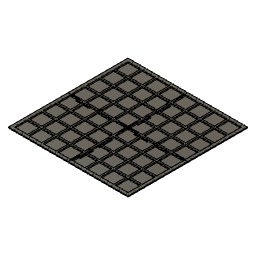
šachovnice v5 v1 (Autodesk Fusion 360 design; units mm, degrees)
Autodesk Fusion 360 part; units mm, degrees
sketch "Sketch1" plane through (0, 0, 0) normal (0, 0, 1) x (1, 0, 0)
  line L0 (-146.9, 146.9) -> (146.9, 146.9)
  line L1 (146.9, 146.9) -> (146.9, -146.9)
  line L2 (146.9, -146.9) -> (-146.9, -146.9)
  line L3 (-146.9, -146.9) -> (-146.9, 146.9)
  line L4 (-111.9, 146.9) -> (-111.9, -146.9) construction
  line L5 (-146.9, 111.9) -> (146.9, 111.9) construction
  line L6 (-74.6, 146.9) -> (-74.6, -146.9) construction
  line L7 (-37.3, 146.9) -> (-37.3, -146.9) construction
  line L8 (0, 146.9) -> (0, -146.9) construction
  line L9 (37.3, 146.9) -> (37.3, -146.9) construction
  line L10 (74.6, 146.9) -> (74.6, -146.9) construction
  line L11 (111.9, 146.9) -> (111.9, -146.9) construction
  line L12 (-146.9, 74.6) -> (146.9, 74.6) construction
  line L13 (-146.9, 37.3) -> (146.9, 37.3) construction
  line L14 (-146.9, 0) -> (146.9, 0) construction
  line L15 (-146.9, -37.3) -> (146.9, -37.3) construction
  line L16 (-146.9, -74.6) -> (146.9, -74.6) construction
  line L17 (-146.9, -111.9) -> (146.9, -111.9) construction
  line L18 (-113.9, 146.9) -> (-113.9, -146.9)
  line L19 (-76.6, 146.9) -> (-76.6, -146.9)
  line L20 (-39.3, 146.9) -> (-39.3, -146.9)
  line L21 (-2, 146.9) -> (-2, -146.9)
  line L22 (35.3, 146.9) -> (35.3, -146.9)
  line L23 (72.6, 146.9) -> (72.6, -146.9)
  line L24 (109.9, 146.9) -> (109.9, -146.9)
  line L25 (-146.9, 109.9) -> (146.9, 109.9)
  line L26 (-146.9, 113.9) -> (146.9, 113.9)
  line L27 (-109.9, 146.9) -> (-109.9, -146.9)
  line L28 (-72.6, 146.9) -> (-72.6, -146.9)
  line L29 (-35.3, 146.9) -> (-35.3, -146.9)
  line L30 (2, 146.9) -> (2, -146.9)
  line L31 (39.3, 146.9) -> (39.3, -146.9)
  line L32 (76.6, 146.9) -> (76.6, -146.9)
  line L33 (113.9, 146.9) -> (113.9, -146.9)
  line L34 (-146.9, 76.6) -> (146.9, 76.6)
  line L35 (-146.9, 72.6) -> (146.9, 72.6)
  line L36 (-146.9, 39.3) -> (146.9, 39.3)
  line L37 (-146.9, 35.3) -> (146.9, 35.3)
  line L38 (-146.9, 2) -> (146.9, 2)
  line L39 (-146.9, -2) -> (146.9, -2)
  line L40 (-146.9, -35.3) -> (146.9, -35.3)
  line L41 (-146.9, -39.3) -> (146.9, -39.3)
  line L42 (-146.9, -72.6) -> (146.9, -72.6)
  line L43 (-146.9, -76.6) -> (146.9, -76.6)
  line L44 (-146.9, -109.9) -> (146.9, -109.9)
  line L45 (-146.9, -113.9) -> (146.9, -113.9)
  line L46 (150.9, -150.9) -> (-150.9, -150.9)
  line L47 (-150.9, -150.9) -> (-150.9, 150.9)
  line L48 (-150.9, 150.9) -> (150.9, 150.9)
  line L49 (150.9, 150.9) -> (150.9, -150.9)
  line L50 (-154.9, -154.9) -> (-154.9, 154.9)
  line L51 (-154.9, 154.9) -> (154.9, 154.9)
  line L52 (154.9, 154.9) -> (154.9, -154.9)
  line L53 (154.9, -154.9) -> (-154.9, -154.9)
  dimension "d8" = 37.3
  dimension "d9" = 0
  dimension "d14" = 0
  dimension "d15" = -37.3
  dimension "d21" = -8
  dimension "d30" = 2
  dimension "d31" = -2
  dimension "d32" = 2
  dimension "d33" = -2
  dimension "d35" = 35
  dimension "d36" = 35
  constraint horizontal L0
  constraint vertical L1
  constraint horizontal L2
  constraint vertical L3
  constraint equal L0 L3
  constraint coincident L0 L4.start
  constraint coincident L2 L4.end
  constraint perpendicular L2 L4
  constraint coincident L3 L5.start
  constraint coincident L1 L5.end
  constraint perpendicular L1 L5
  constraint midpoint L8 origin
  constraint coincident L1 L26.end
  constraint coincident L1 L25.end
  constraint coincident L3 L26.start
  constraint coincident L3 L25.start
  constraint coincident L0 L18.start
  constraint coincident L0 L27.start
  constraint coincident L14 origin
  constraint coincident L8 origin
  measures "d35" distance of L3 L4
  measures "d36" distance of L0 L5
extrude "Extrude1" add sketch "Sketch1" along normal blind 4 contours L0 L18 L26 L27 | L3 L18 L25 L26 | L18 L25 L26 L27 | L0 L19 L26 L28 | L19 L25 L26 L27 | L18 L25 L27 L34 | L3 L18 L34 L35 | L19 L25 L26 L28 | L18 L27 L34 L35 | L0 L20 L26 L29 | L20 L25 L26 L28 | L19 L25 L28 L34 | L19 L27 L34 L35 | L18 L27 L35 L36 | L3 L18 L36 L37 | L20 L25 L26 L29 | L19 L28 L34 L35 | L18 L27 L36 L37 | L0 L21 L26 L30 | L21 L25 L26 L29 | L20 L25 L29 L34 | L20 L28 L34 L35 | L19 L28 L35 L36 | L19 L27 L36 L37 | L18 L27 L37 L38 | L3 L18 L38 L39 | L21 L25 L26 L30 | L20 L29 L34 L35 | L19 L28 L36 L37 | L18 L27 L38 L39 | L0 L22 L26 L31 | L22 L25 L26 L30 | L21 L25 L30 L34 | L21 L29 L34 L35 | L20 L29 L35 L36 | L20 L28 L36 L37 | L19 L28 L37 L38 | L19 L27 L38 L39 | L18 L27 L39 L40 | L3 L18 L40 L41 | L22 L25 L26 L31 | L21 L30 L34 L35 | L20 L29 L36 L37 | L19 L28 L38 L39 | L18 L27 L40 L41 | L0 L23 L26 L32 | L23 L25 L26 L31 | L22 L25 L31 L34 | L22 L30 L34 L35 | L21 L30 L35 L36 | L21 L29 L36 L37 | L20 L29 L37 L38 | L20 L28 L38 L39 | L19 L28 L39 L40 | L19 L27 L40 L41 | L18 L27 L41 L42 | L3 L18 L42 L43 | L23 L25 L26 L32 | L22 L31 L34 L35 | L21 L30 L36 L37 | L20 L29 L38 L39 | L19 L28 L40 L41 | L18 L27 L42 L43 | L0 L24 L26 L33 | L24 L25 L26 L32 | L23 L25 L32 L34 | L23 L31 L34 L35 | L22 L31 L35 L36 | L22 L30 L36 L37 | L21 L30 L37 L38 | L21 L29 L38 L39 | L20 L29 L39 L40 | L20 L28 L40 L41 | L19 L28 L41 L42 | L19 L27 L42 L43 | L18 L27 L43 L44 | L3 L18 L44 L45 | L24 L25 L26 L33 | L23 L32 L34 L35 | L22 L31 L36 L37 | L21 L30 L38 L39 | L20 L29 L40 L41 | L19 L28 L42 L43 | L18 L27 L44 L45 | L1 L25 L26 L33 | L24 L25 L33 L34 | L24 L32 L34 L35 | L23 L32 L35 L36 | L23 L31 L36 L37 | L22 L31 L37 L38 | L22 L30 L38 L39 | L21 L30 L39 L40 | L21 L29 L40 L41 | L20 L29 L41 L42 | L20 L28 L42 L43 | L19 L28 L43 L44 | L19 L27 L44 L45 | L2 L18 L27 L45 | L24 L33 L34 L35 | L23 L32 L36 L37 | L22 L31 L38 L39 | L21 L30 L40 L41 | L20 L29 L42 L43 | L19 L28 L44 L45 | L1 L33 L34 L35 | L24 L33 L35 L36 | L24 L32 L36 L37 | L23 L32 L37 L38 | L23 L31 L38 L39 | L22 L31 L39 L40 | L22 L30 L40 L41 | L21 L30 L41 L42 | L21 L29 L42 L43 | L20 L29 L43 L44 | L20 L28 L44 L45 | L2 L19 L28 L45 | L24 L33 L36 L37 | L23 L32 L38 L39 | L22 L31 L40 L41 | L21 L30 L42 L43 | L20 L29 L44 L45 | L1 L33 L36 L37 | L24 L33 L37 L38 | L24 L32 L38 L39 | L23 L32 L39 L40 | L23 L31 L40 L41 | L22 L31 L41 L42 | L22 L30 L42 L43 | L21 L30 L43 L44 | L21 L29 L44 L45 | L2 L20 L29 L45 | L24 L33 L38 L39 | L23 L32 L40 L41 | L22 L31 L42 L43 | L21 L30 L44 L45 | L1 L33 L38 L39 | L24 L33 L39 L40 | L24 L32 L40 L41 | L23 L32 L41 L42 | L23 L31 L42 L43 | L22 L31 L43 L44 | L22 L30 L44 L45 | L2 L21 L30 L45 | L24 L33 L40 L41 | L23 L32 L42 L43 | L22 L31 L44 L45 | L1 L33 L40 L41 | L24 L33 L41 L42 | L24 L32 L42 L43 | L23 L32 L43 L44 | L23 L31 L44 L45 | L2 L22 L31 L45 | L24 L33 L42 L43 | L23 L32 L44 L45 | L1 L33 L42 L43 | L24 L33 L43 L44 | L24 L32 L44 L45 | L2 L23 L32 L45 | L24 L33 L44 L45 | L1 L33 L44 L45 | L2 L24 L33 L45 | L46 L47 L48 L49 | L50 L51 L52 L53 makes body 1
extrude "Extrude2" add sketch "Sketch1" along normal blind 1 contours L0 L3 L18 L26 | L0 L19 L26 L27 | L3 L18 L25 L34 | L0 L20 L26 L28 | L19 L25 L27 L34 | L3 L18 L35 L36 | L0 L21 L26 L29 | L20 L25 L28 L34 | L19 L27 L35 L36 | L3 L18 L37 L38 | L0 L22 L26 L30 | L21 L25 L29 L34 | L20 L28 L35 L36 | L19 L27 L37 L38 | L3 L18 L39 L40 | L0 L23 L26 L31 | L22 L25 L30 L34 | L21 L29 L35 L36 | L20 L28 L37 L38 | L19 L27 L39 L40 | L3 L18 L41 L42 | L0 L24 L26 L32 | L23 L25 L31 L34 | L22 L30 L35 L36 | L21 L29 L37 L38 | L20 L28 L39 L40 | L19 L27 L41 L42 | L3 L18 L43 L44 | L0 L1 L26 L33 | L24 L25 L32 L34 | L23 L31 L35 L36 | L22 L30 L37 L38 | L21 L29 L39 L40 | L20 L28 L41 L42 | L19 L27 L43 L44 | L2 L3 L18 L45 | L1 L25 L33 L34 | L24 L32 L35 L36 | L23 L31 L37 L38 | L22 L30 L39 L40 | L21 L29 L41 L42 | L20 L28 L43 L44 | L2 L19 L27 L45 | L1 L33 L35 L36 | L24 L32 L37 L38 | L23 L31 L39 L40 | L22 L30 L41 L42 | L21 L29 L43 L44 | L2 L20 L28 L45 | L1 L33 L37 L38 | L24 L32 L39 L40 | L23 L31 L41 L42 | L22 L30 L43 L44 | L2 L21 L29 L45 | L1 L33 L39 L40 | L24 L32 L41 L42 | L23 L31 L43 L44 | L2 L22 L30 L45 | L1 L33 L41 L42 | L24 L32 L43 L44 | L2 L23 L31 L45 | L1 L33 L43 L44 | L2 L24 L32 L45 | L1 L2 L33 L45 bodies 1
extrude "Extrude3" cut sketch "Sketch1" along normal blind 2 contours L50 L51 L52 L53 bodies 1
sketch "Sketch2" plane through (0, 0, 0) normal (0, 0, -1) x (1, 0, 0)
  line L0 (-150.9, 150.9) -> (-150.9, -150.9)
  line L1 (-150.9, -150.9) -> (150.9, -150.9)
  line L2 (150.9, -150.9) -> (150.9, 150.9)
  line L3 (150.9, 150.9) -> (-150.9, 150.9)
sketch "Sketch3" plane through (0, 0, 0) normal (0, 0, 1) x (-1, 0, 0)
  line L0 (154.9, -154.9) -> (154.9, 154.9)
  line L1 (-5, -105.4443) -> (-5, -70) construction
  line L2 (5, -130.4443) -> (5, -95.4443) construction
  line L3 (0, -125.4443) -> (5, -130.4443) construction
  line L4 (-5, -55) -> (-5, -20) construction
  line L5 (5, -80) -> (5, -45) construction
  line L6 (-5, 45) -> (-5, 80) construction
  line L7 (5, 20) -> (5, 55) construction
  line L8 (-5, 130) -> (0, 125) construction
  line L9 (-5, 95) -> (-5, 130) construction
  line L10 (5, 70) -> (5, 105) construction
  line L11 (5.1, -130.6857) -> (5.1, -95.2029)
  line L12 (-4.9, -105.2029) -> (-4.9, -70.2414)
  line L13 (5.1, -80.2414) -> (5.1, -44.7586)
  line L14 (-4.9, -54.7586) -> (-4.9, -20.2414)
  line L15 (5.1, 19.7586) -> (5.1, 55.2414)
  line L16 (-4.9, 45.2414) -> (-4.9, 79.7586)
  line L17 (5.1, 69.7586) -> (5.1, 105.2414)
  line L18 (-4.9, 95.2414) -> (-4.9, 129.7586)
  line L19 (4.9, -130.2029) -> (4.9, -95.6857)
  line L20 (-5.1, -105.6857) -> (-5.1, -69.7586)
  line L21 (4.9, -79.7586) -> (4.9, -45.2414)
  line L22 (-5.1, -55.2414) -> (-5.1, -19.7586)
  line L23 (4.9, 20.2414) -> (4.9, 54.7586)
  line L24 (-5.1, 44.7586) -> (-5.1, 80.2414)
  line L25 (4.9, 70.2414) -> (4.9, 104.7586)
  line L26 (-5.1, 94.7586) -> (-5.1, 130.2414)
  line L27 (55, -5) -> (20, -5) construction
  line L28 (79.7586, 4.9) -> (45.2414, 4.9)
  line L29 (80, 5) -> (45, 5) construction
  line L30 (-44.7586, -5.1) -> (-80.2414, -5.1)
  line L31 (-95.0618, -4.9) -> (-129.5789, -4.9)
  line L32 (-45.2414, -4.9) -> (-79.7586, -4.9)
  line L33 (80.2414, 5.1) -> (44.7586, 5.1)
  line L34 (130.2414, 5.1) -> (94.7586, 5.1)
  line L35 (-19.7586, 5.1) -> (-55.2414, 5.1)
  line L36 (-20, 5) -> (-55, 5) construction
  line L37 (105, -5) -> (70, -5) construction
  line L38 (54.7586, -4.9) -> (20.2414, -4.9)
  line L39 (55.2414, -5.1) -> (19.7586, -5.1)
  line L40 (-20.2414, 4.9) -> (-54.7586, 4.9)
  line L41 (105.2414, -5.1) -> (69.7586, -5.1)
  line L42 (-94.8203, -5) -> (-129.8203, -5) construction
  line L43 (104.7586, -4.9) -> (70.2414, -4.9)
  line L44 (130, 5) -> (95, 5) construction
  line L45 (-45, -5) -> (-80, -5) construction
  line L46 (-69.6687, 5.1898) -> (-105.1516, 5.1898)
  line L47 (-94.5789, -5.1) -> (-130.0618, -5.1)
  line L48 (-70.1516, 4.9898) -> (-104.6687, 4.9898)
  line L49 (-69.9102, 5.0898) -> (-104.9102, 5.0898) construction
  line L50 (129.7586, 4.9) -> (95.2414, 4.9)
  line L51 (-129.8203, -5) -> (-124.8203, 0) construction
  line L52 (20, -5) -> (25, 0) construction
  line L53 (19.7586, -5.1) -> (24.7586, -0.1)
  line L54 (25, 0) -> (0, 0) construction
  line L55 (25.2414, 0.1) -> (0, 0.1)
  line L56 (24.7586, -0.1) -> (0, -0.1)
  line L57 (-20, 5) -> (-25, 0) construction
  line L58 (-19.7586, 5.1) -> (-24.7586, 0.1)
  line L59 (-24.7586, 0.1) -> (0, 0.1)
  line L60 (-25, 0) -> (0, 0) construction
  line L61 (-20.2414, 4.9) -> (-25.2414, -0.1)
  line L62 (0, -0.1) -> (-25.2414, -0.1)
  line L63 (-5, -20) -> (0, -25) construction
  line L64 (0, -25) -> (0, 0) construction
  line L65 (-5.1, -19.7586) -> (-0.1, -24.7586)
  line L66 (-0.1, -24.7586) -> (-0.1, -0.1)
  line L67 (-4.9, -20.2414) -> (0.1, -25.2414)
  line L68 (0.1, -25.2414) -> (0.1, -0.1)
  line L69 (5, 20) -> (0, 25) construction
  line L70 (0, 25) -> (0, 0) construction
  line L71 (5.1, 19.7586) -> (0.1, 24.7586)
  line L72 (0.1, 24.7586) -> (0.1, 0.1)
  line L73 (4.9, 20.2414) -> (-0.1, 25.2414)
  line L74 (-0.1, 25.2414) -> (-0.1, 0.1)
  line L75 (-124.8203, 0) -> (-157, 0) construction
  line L76 (-124.5789, 0.1) -> (-157, 0.1)
  line L77 (-130.0618, -5.1) -> (-125.0618, -0.1)
  line L78 (-125.0618, -0.1) -> (-157, -0.1)
  line L79 (0, 125) -> (0, 163.2119) construction
  line L80 (-5.1, 130.2414) -> (-0.1, 125.2414)
  line L81 (-0.1, 125.2414) -> (-0.1, 156.7338)
  line L82 (0.1, 124.7586) -> (0.1, 159.9994)
  line L83 (130, 5) -> (125, 0) construction
  line L84 (125, 0) -> (175, 0) construction
  line L85 (130.2414, 5.1) -> (125.2414, 0.1)
  line L86 (125.2414, 0.1) -> (175.0792, 0.1)
  line L87 (129.7586, 4.9) -> (124.7586, -0.1)
  line L88 (124.7586, -0.1) -> (175.0791, -0.1)
  line L89 (0, -125.4443) -> (0, -160) construction
  line L90 (-0.1, -125.2029) -> (-0.1, -160)
  line L91 (5.1, -130.6857) -> (0.1, -125.6857)
  line L92 (0.1, -125.6857) -> (0.1, -160)
  line L93 (5.1, 55.2414) -> (-4.9, 45.2414)
  line L94 (4.9, 54.7586) -> (-5.1, 44.7586)
  line L95 (5, 55) -> (-5, 45) construction
  line L96 (5, 70) -> (-5, 80) construction
  line L97 (4.9, 70.2414) -> (-5.1, 80.2414)
  line L98 (5.1, 69.7586) -> (-4.9, 79.7586)
  line L99 (4.9, 104.7586) -> (-5.1, 94.7586)
  line L100 (5, 105) -> (-5, 95) construction
  line L101 (5.1, 105.2414) -> (-4.9, 95.2414)
  line L102 (0.1, 124.7586) -> (-4.9, 129.7586)
  line L103 (-55, 5) -> (-45, -5) construction
  line L104 (-45.2414, -4.9) -> (-55.2414, 5.1)
  line L105 (-54.7586, 4.9) -> (-44.7586, -5.1)
  line L106 (-69.9102, 5.0898) -> (-80, -5) construction
  line L107 (-70.1516, 4.9898) -> (-80.2414, -5.1)
  line L108 (-69.6687, 5.1898) -> (-79.7586, -4.9)
  line L109 (-94.8203, -5) -> (-104.9102, 5.0898) construction
  line L110 (-105.1516, 5.1898) -> (-95.0618, -4.9)
  line L111 (-104.6687, 4.9898) -> (-94.5789, -5.1)
  line L112 (-124.5789, 0.1) -> (-129.5789, -4.9)
  line L113 (5, -45) -> (-5, -55) construction
  line L114 (4.9, -45.2414) -> (-5.1, -55.2414)
  line L115 (5.1, -44.7586) -> (-4.9, -54.7586)
  line L116 (5, -80) -> (-5, -70) construction
  line L117 (4.9, -79.7586) -> (-5.1, -69.7586)
  line L118 (5.1, -80.2414) -> (-4.9, -70.2414)
  line L119 (4.9, -95.6857) -> (-5.1, -105.6857)
  line L120 (-5, -105.4443) -> (5, -95.4443) construction
  line L121 (5.1, -95.2029) -> (-4.9, -105.2029)
  line L122 (4.9, -130.2029) -> (-0.1, -125.2029)
  line L123 (25.2414, 0.1) -> (20.2414, -4.9)
  line L124 (45.2414, 4.9) -> (55.2414, -5.1)
  line L125 (55, -5) -> (45, 5) construction
  line L126 (54.7586, -4.9) -> (44.7586, 5.1)
  line L127 (80.2414, 5.1) -> (70.2414, -4.9)
  line L128 (80, 5) -> (70, -5) construction
  line L129 (79.7586, 4.9) -> (69.7586, -5.1)
  line L130 (95.2414, 4.9) -> (105.2414, -5.1)
  line L131 (95, 5) -> (105, -5) construction
  line L132 (104.7586, -4.9) -> (94.7586, 5.1)
  line L133 (-157, 0.1) -> (-157, -0.1)
  line L134 (0.1, 159.9994) -> (-0.1, 156.7338)
  line L135 (175.0791, -0.1) -> (175.0792, 0.1)
  line L136 (0.1, -160) -> (-0.1, -160)
  dimension "d67" = 0.2
  dimension "d68" = 0.1
  dimension "d69" = 45
  dimension "d70" = 0.1
  dimension "d71" = 5
  dimension "d72" = 0.1
  dimension "d74" = 45
  dimension "d75" = 0.1
  dimension "d76" = 10
  dimension "d77" = 0.1
  dimension "d78" = 35
  dimension "d79" = 25
  dimension "d80" = 45
  dimension "d81" = 0.1
  dimension "d82" = 45
  dimension "d83" = 0.1
  dimension "d84" = 10
  dimension "d85" = 35
  dimension "d86" = 35
  dimension "d87" = 45
  dimension "d88" = 0.1
  dimension "d90" = 45
  dimension "d91" = 0.1
  dimension "d92" = 45
  dimension "d93" = 0.1
  dimension "d97" = 45
  dimension "d99" = 5
  dimension "d100" = 0.1
  dimension "d102" = 0.1
  dimension "d103" = 0.1
  dimension "d104" = 45
  dimension "d105" = 0.1
  dimension "d106" = 45
  dimension "d107" = 35
  dimension "d108" = 5
  dimension "d109" = 25
  dimension "d110" = 0.1
  dimension "d111" = 45
  dimension "d112" = 45
  dimension "d113" = 0.1
  dimension "d114" = 35
  dimension "d115" = 10
  dimension "d116" = 0.1
  dimension "d117" = 45
  dimension "d118" = 45
  dimension "d119" = 0.1
  dimension "d121" = 45
  dimension "d122" = 45
  dimension "d123" = 0.1
  dimension "d124" = 10.0898
  dimension "d125" = 10.0898
  dimension "d126" = 0.1
  dimension "d127" = 35
  dimension "d128" = 35
  dimension "d129" = 45
  dimension "d130" = 45
  dimension "d131" = 0.1
  dimension "d132" = 0.1
  dimension "d133" = 5
  dimension "d134" = 35
  dimension "d135" = 0.1
  dimension "d136" = 45
  dimension "d137" = 45
  dimension "d138" = 0.1
  dimension "d139" = 25
  dimension "d141" = 0.1
  dimension "d142" = 35
  dimension "d143" = 5
  dimension "d145" = 45
  dimension "d146" = 0.1
  dimension "d147" = 45
  dimension "d148" = 0.1
  dimension "d149" = 35
  dimension "d150" = 10
  dimension "d151" = 45
  dimension "d152" = 45
  dimension "d153" = 0.1
  dimension "d154" = 0.1
  dimension "d155" = 45
  dimension "d156" = 45
  dimension "d158" = 0.1
  dimension "d159" = 35.4443
  dimension "d160" = 35
  dimension "d161" = 10
  dimension "d164" = 0.1
  dimension "d165" = 10
  dimension "d166" = 45
  dimension "d167" = 45
  dimension "d168" = 0.1
  dimension "d169" = 0.1
  dimension "d170" = 5
  dimension "d171" = 25
  dimension "d172" = 45
  dimension "d173" = 45
  dimension "d174" = 5
  dimension "d176" = 0.1
  dimension "d178" = 0.1
  dimension "d179" = 45
  dimension "d180" = 45
  dimension "d181" = 10
  dimension "d182" = 0.1
  dimension "d183" = 35
  dimension "d184" = 35
  dimension "d185" = 0.1
  dimension "d186" = 45
  dimension "d187" = 45
  dimension "d188" = 10
  dimension "d189" = 35
  dimension "d190" = 0.1
  dimension "d191" = 0.1
  dimension "d192" = 45
  dimension "d193" = 45
  dimension "d194" = 10
  dimension "d195" = 0.1
  dimension "d196" = 35
  dimension "d198" = 0.1
  dimension "d199" = 45
  dimension "d200" = 0.1
  dimension "d201" = 5
  dimension "d202" = 0.1
  constraint parallel L52 L53
  constraint coincident L54.end L60.end
  constraint horizontal L55
  constraint parallel L54 L56
  constraint parallel L59 L60
  constraint parallel L57 L58
  constraint parallel L57 L61
  constraint parallel L60 L62
  constraint perpendicular L60 L64
  constraint coincident L62 L66.end
  constraint perpendicular L62 L66
  constraint parallel L65 L67
  constraint coincident L56 L68.end
  constraint perpendicular L56 L68
  constraint coincident L55 L72.end
  constraint perpendicular L55 L72
  constraint coincident L59 L74.end
  constraint perpendicular L59 L74
  constraint parallel L70 L74
  constraint parallel L75 L76
  constraint parallel L47 L78
  constraint parallel L44 L84
  constraint parallel L34 L86
  constraint parallel L83 L87
  constraint parallel L50 L88
  constraint parallel L99 L101
  constraint equal L95 L100
  constraint parallel L8 L102
  constraint parallel L79 L82
  constraint parallel L36 L40
  constraint parallel L103 L105
  constraint parallel L32 L45
  constraint parallel L106 L107
  constraint parallel L46 L49
  constraint parallel L109 L111
  constraint parallel L51 L77
  constraint parallel L4 L14
  constraint parallel L114 L115
  constraint parallel L5 L13
  constraint parallel L116 L117
  constraint parallel L1 L12
  constraint parallel L120 L121
  constraint parallel L2 L19
  constraint parallel L3 L122
  constraint parallel L89 L90
  constraint parallel L27 L38
  constraint parallel L124 L125
  constraint parallel L29 L33
  constraint parallel L128 L129
  constraint parallel L37 L43
  constraint parallel L130 L132
  constraint parallel L34 L44
  constraint parallel L83 L85
  constraint perpendicular L78 L133
  constraint perpendicular L90 L136
  measures "d67" distance of L72 L74
  measures "d68" distance of L70 L72
  measures "d69" angle of L69 L70
  measures "d70" distance of L69 L71
  measures "d71" distance of L7 L70
  measures "d72" distance of L7 L15
  measures "d74" angle of L7 L95
  measures "d75" distance of L94 L95
  measures "d76" distance of L6 L7
  measures "d77" distance of L6 L16
  measures "d78" distance of L7.end L7.start
  measures "d79" distance of L54.end L69.end
  measures "d80" angle of L6 L96
  measures "d81" distance of L96 L98
  measures "d82" angle of L10 L96
  measures "d83" distance of L10 L17
  measures "d84" distance of L6 L10
  measures "d85" distance of L10.end L10.start
  measures "d86" distance of L6.end L6.start
  measures "d87" angle of L10 L100
  measures "d88" distance of L99 L100
  measures "d90" angle of L9 L100
  measures "d91" distance of L9 L18
  measures "d92" angle of L8 L9
  measures "d93" distance of L8 L102
  measures "d97" angle of L8 L79
  measures "d99" distance of L9 L79
  measures "d100" distance of L79 L82
  measures "d102" distance of L59 L60
  measures "d103" distance of L57 L58
  measures "d104" angle of L57 L60
  measures "d105" distance of L36 L40
  measures "d106" angle of L36 L57
  measures "d107" distance of L36.start L36.end
  measures "d108" distance of L36 L60
  measures "d109" distance of L57.end L54.end
  measures "d110" distance of L103 L105
  measures "d111" angle of L45 L103
  measures "d112" angle of L36 L103
  measures "d113" distance of L32 L45
  measures "d114" distance of L45.end L45.start
  measures "d115" distance of L36 L45
  measures "d116" distance of L106 L108
  measures "d117" angle of L45 L106
  measures "d118" angle of L49 L106
  measures "d119" distance of L46 L49
  measures "d121" angle of L49 L109
  measures "d122" angle of L42 L109
  measures "d123" distance of L109 L111
  measures "d124" distance of L42 L49
  measures "d125" distance of L45 L49
  measures "d126" distance of L31 L42
  measures "d127" distance of L49.start L49.end
  measures "d128" distance of L8.start L9.start
  measures "d129" angle of L42 L51
  measures "d130" angle of L51 L75
  measures "d131" distance of L51 L112
  measures "d132" distance of L75 L76
  measures "d133" distance of L42 L75
  measures "d134" distance of L42.start L42.end
  measures "d135" distance of L64 L68
  measures "d136" angle of L63 L64
  measures "d137" angle of L4 L63
  measures "d138" distance of L63 L65
  measures "d139" distance of L63.end L54.end
  measures "d141" distance of L4 L14
  measures "d142" distance of L4.end L4.start
  measures "d143" distance of L4 L64
  measures "d145" angle of L4 L113
  measures "d146" distance of L113 L114
  measures "d147" angle of L5 L113
  measures "d148" distance of L5 L13
  measures "d149" distance of L5.end L5.start
  measures "d150" distance of L4 L5
  measures "d151" angle of L5 L116
  measures "d152" angle of L1 L116
  measures "d153" distance of L116 L117
  measures "d154" distance of L1 L12
  measures "d155" angle of L1 L120
  measures "d156" angle of L2 L120
  measures "d158" distance of L120 L121
  measures "d159" distance of L1.end L1.start
  measures "d160" distance of L2.end L2.start
  measures "d161" distance of L1 L2
  measures "d164" distance of L2 L11
  measures "d165" distance of L1 L5
  measures "d166" angle of L2 L3
  measures "d167" angle of L3 L89
  measures "d168" distance of L3 L91
  measures "d169" distance of L89 L92
  measures "d170" distance of L2 L89
  measures "d171" distance of L52.end L54.end
  measures "d172" angle of L52 L54
  measures "d173" angle of L27 L52
  measures "d174" distance of L27 L54
  measures "d176" distance of L52 L123
  measures "d178" distance of L27 L38
  measures "d179" angle of L27 L125
  measures "d180" angle of L29 L125
  measures "d181" distance of L27 L29
  measures "d182" distance of L124 L125
  measures "d183" distance of L29.end L29.start
  measures "d184" distance of L27.start L27.end
  measures "d185" distance of L29 L33
  measures "d186" angle of L29 L128
  measures "d187" angle of L37 L128
  measures "d188" distance of L29 L37
  measures "d189" distance of L37.start L37.end
  measures "d190" distance of L127 L128
  measures "d191" distance of L37 L43
  measures "d192" angle of L37 L131
  measures "d193" angle of L44 L131
  measures "d194" distance of L37 L44
  measures "d195" distance of L131 L132
  measures "d196" distance of L44.end L44.start
  measures "d198" distance of L34 L44
  measures "d199" angle of L44 L83
  measures "d200" distance of L83 L85
  measures "d201" distance of L44 L84
  measures "d202" distance of L84 L86
extrude "Extrude5" cut sketch "Sketch3" along normal through all contours L0 L28 L30 L31 L32 L33 L34 L35 L38 L39 L40 L41 L43 L46 L47 L48 L50 L53 L55 L56 L58 L59 L61 L62 L76 L77 L78 L85 L86 L87 L88 L104 L105 L107 L108 L110 L111 L112 L123 L124 L126 L127 L129 L130 L132 L133 | L11 L12 L13 L14 L19 L20 L21 L22 L56 L62 L65 L66 L67 L68 L90 L91 L92 L114 L115 L117 L118 L119 L121 L122 L136 | L15 L16 L17 L18 L23 L24 L25 L26 L55 L59 L71 L72 L73 L74 L80 L81 L82 L93 L94 L97 L98 L99 L101 L102 L134 bodies 1 makes body 2 at (-87.0805, 83.7343, 0) makes body 3 at (-83.5862, -87.0805, 0) makes body 4 at (83.5263, 87.2286, 0)
